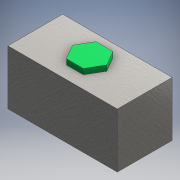
# Autodesk Inventor part: Basic Sensor
Saved by Autodesk Inventor 2016 (Build 200138000, 138)
## iProperties
Created: 2016-02-23
Part Number: Basic Sensor
Material: Generic
Document SubType Name: Modeling
Designer: Kenneth Daniel
Density: 1 g/cm^3
Appearance: Default
Author: Kenneth Daniel
Autodesk Inventor part; units mm, degrees
ref_plane "YZ Plane" through (0, 0, 0) normal (1, 0, 0) x (0, 1, 0)
ref_plane "XZ Plane" through (0, 0, 0) normal (0, 1, 0) x (-1, 0, 0)
ref_plane "XY Plane" through (0, 0, 0) normal (0, 0, 1) x (1, 0, 0)
sketch "Sketch1" plane through (0, 0, 0) normal (0, 0, 1) x (1, 0, 0)
  line L0 (0, 0) -> (20, 0)
  line L1 (20, 0) -> (20, 10)
  line L2 (20, 10) -> (0, 10)
  line L3 (0, 10) -> (0, 0)
  dimension "d0" = 20
  dimension "d1" = 10
  constraints: 8 end point, 2 parallel, 1 horizontal, 1 perpendicular
  measures "d0" distance of L0.start L0.end
  measures "d1" distance of L1.end L0.end
extrude "Extrusion1" add sketch "Sketch1" along normal blind 10
sketch "Sketch2" plane through (0, 0, 10) normal (0, 0, 1) x (1, 0, 0)
  line L0 (0, 10) -> (0, 0) construction
  line L1 (0, 0) -> (19.8824, 10) construction
  line L2 (0, 10) -> (19.8824, 0) construction
  line L3 (6.8271, 5) -> (8.3842, 7.6969)
  line L4 (8.3842, 7.6969) -> (11.4983, 7.6969)
  line L5 (11.4983, 7.6969) -> (13.0553, 5)
  line L6 (13.0553, 5) -> (11.4983, 2.3031)
  line L7 (11.4983, 2.3031) -> (8.3842, 2.3031)
  line L8 (8.3842, 2.3031) -> (6.8271, 5)
  point P0 (9.9412, 5)
  constraints: 16 end point, 1 midpoint, 13 other
extrude "Extrusion2" add sketch "Sketch2" along normal blind 1
body "Solid1"
